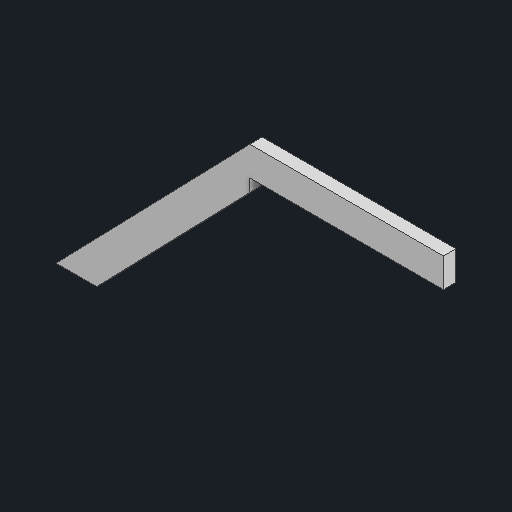
# Autodesk Inventor part: side-side1
Saved by Autodesk Inventor 2026 (Build 300175000, 175)
## iProperties
Created: 2024-09-20
Part Number: side-side1
Material: Generic
Document SubType Name: Modeling
Designer: User
Density: 1 g/cm^3
Appearance: Default
Author: User
Autodesk Inventor part; units mm, degrees
ref_plane "YZ Plane" through (0, 0, 0) normal (1, 0, 0) x (0, 1, 0)
ref_plane "XZ Plane" through (0, 0, 0) normal (0, 1, 0) x (-1, 0, 0)
ref_plane "XY Plane" through (0, 0, 0) normal (0, 0, 1) x (1, 0, 0)
sketch "Sketch1" plane through (0, 0, 0) normal (0, 0, 1) x (1, 0, 0)
  line L0 (0, 0) -> (1219.2, 0) projected
  line L1 (1181.1, 0) -> (1181.1, 609.6) projected
  line L2 (1181.1, 1219.2) -> (0, 0) projected
  line L3 (0, 0) -> (590.55, 609.6)
  line L4 (590.55, 520.7) -> (590.55, 481.8325)
  line L5 (590.55, 481.8325) -> (123.7747, 0)
  line L6 (590.55, 609.6) -> (1181.1, 609.6)
  line L7 (1181.1, 520.7) -> (590.55, 520.7)
  dimension "d0" = 88.9
  dimension "d1" = 88.9
  constraints: 10 end point, 2 point on line, 1 horizontal, 1 midpoint, 1 parallel, 1 perpendicular, 1 vertical
  measures "d0" distance between parallel lines of L2 L5
  measures "d1" distance between parallel lines of L6 L7
extrude "Extrusion1" add sketch "Sketch1" against normal blind 38.1 contours L2 L6 L1 L7 L4 L5 L0
body "Solid1"
